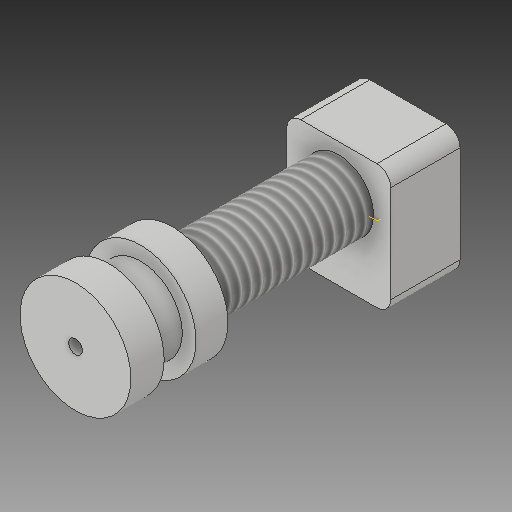
# Autodesk Inventor part: Hotend Mock Up
Saved by Autodesk Inventor 2018 (Build 220112000, 112)
## iProperties
Created: 2016-06-25
Part Number: Hotend Mock Up
Material: Generic
Document SubType Name: Modeling
Designer: joshm
Density: 1 g/cm^3
Appearance: Default
Mass: 6.93473 g
Surface Area: 30.5919 cm^2
Volume: 6.93473 cm^3
Author: joshm
Autodesk Inventor part; units mm, degrees
ref_plane "YZ Plane" through (0, 0, 0) normal (1, 0, 0) x (0, 1, 0)
ref_plane "XZ Plane" through (0, 0, 0) normal (0, 1, 0) x (-1, 0, 0)
ref_plane "XY Plane" through (0, 0, 0) normal (0, 0, 1) x (1, 0, 0)
sketch "Sketch1" plane through (0, 0, 0) normal (0, 0, 1) x (1, 0, 0)
  arc A0 (10.5041, 10) -> (25.996, 10) centre (18.25, 12) ccw projected
  circle A1 centre (18.25, 12) radius 8
  point P0 (0, 0)
  constraints: 1 centre point, 1 coincident, 1 concentric
extrude "Extrusion1" add sketch "Sketch1" against normal blind 4.8
sketch "Sketch2" plane through (18.25, 12, -4.8) normal (0, 0, -1) x (-1, 0, 0)
  circle A0 centre (0, 0) radius 8 projected
  circle A1 centre (0, 0) radius 6
  point P0 (18.25, -12)
  dimension "d2" = 12
  constraints: 1 centre point, 1 coincident
  measures "d2" diameter of A1
extrude "Extrusion2" add sketch "Sketch2" along normal blind 4.6 contours A1
sketch "Sketch3" plane through (18.25, 12, -9.4) normal (0, 0, -1) x (-1, 0, 0)
  circle A0 centre (0, 0) radius 6 projected
  circle A1 centre (0, 0) radius 8
  point P0 (18.25, -12)
  constraints: 1 centre point, 1 coincident
extrude "Extrusion3" add sketch "Sketch3" along normal blind 4.6 contours A0 | A1
sketch "Sketch4" plane through (18.25, 12, -14) normal (0, 0, -1) x (-1, 0, 0)
  circle A0 centre (0, 0) radius 8 projected
  circle A1 centre (0, 0) radius 5
  point P0 (18.25, -12)
  dimension "d7" = 10
  constraints: 1 centre point, 1 coincident
  measures "d7" diameter of A1
extrude "Extrusion4" add sketch "Sketch4" along normal blind 24 contours A1
thread "Thread1" size "M10x1.5" class "6g" standard "ANSI Metric M Profile" full length
sketch "Sketch5" plane through (18.25, 12, -38) normal (0, 0, -1) x (-1, 0, 0)
  line L0 (-5.5007, -11.3783) -> (5.4993, -11.3783)
  line L1 (7.4993, -9.3783) -> (7.4993, 4.6217)
  line L2 (5.4993, 6.6217) -> (-5.5007, 6.6217)
  line L3 (-7.5007, 4.6217) -> (-7.5007, -9.3783)
  line L4 (-7.5007, -11.3783) -> (7.4993, 6.6217) construction
  line L5 (7.4993, -11.3783) -> (-7.5007, 6.6217) construction
  arc A0 (7.4993, 4.6217) -> (5.4993, 6.6217) centre (5.4993, 4.6217) ccw
  arc A1 (-5.5007, 6.6217) -> (-7.5007, 4.6217) centre (-5.5007, 4.6217) ccw
  arc A2 (-7.5007, -9.3783) -> (-5.5007, -11.3783) centre (-5.5007, -9.3783) ccw
  arc A3 (5.4993, -11.3783) -> (7.4993, -9.3783) centre (5.4993, -9.3783) ccw
  point P0 (18.25, -12)
  point P1 (-0.0007, -2.3783)
  dimension "d12" = 15
  dimension "d13" = 18
  dimension "d14" = 2
  constraints: 12 end point, 8 point on circle, 8 point on line, 8 tangent, 4 centre point, 3 equal radius, 2 midpoint, 2 parallel, 1 horizontal, 1 perpendicular
  measures "d12" distance of L5.end L4.end
  measures "d13" distance of L4.end L5.start
  measures "d14" radius of A0
extrude "Extrusion5" add sketch "Sketch5" along normal blind 10
sketch "Sketch6" plane through (18.25, 12, -48) normal (0, 0, -1) x (-1, 0, 0)
  circle A0 centre (0, 0) radius 5 projected
  circle A1 centre (0, 0) radius 1.15
  point P0 (18.25, -12)
  dimension "d17" = 2.3
  constraints: 1 centre point, 1 coincident
  measures "d17" diameter of A1
ref_plane "Work Plane1" through (12.7508, 11.9997, -38) normal (0, 1, 0) x (1, 0, 0)
sketch "Sketch7" plane through (12.7508, 11.9997, -38) normal (0, 1, 0) x (1, 0, 0)
  line L0 (6.6493, 10) -> (4.3493, 10) projected
  line L1 (5.4993, 10) -> (5.4993, 14.106)
  line L2 (5.3539, 14.106) -> (4.3493, 10)
  line L3 (5.4993, 14.106) -> (5.3539, 14.106)
  line L4 (5.4993, 14.106) -> (5.6446, 14.106) construction
  line L5 (5.4993, 10) -> (4.3493, 10)
  line L6 (4.3493, 10) -> (5.3539, 14.106)
  point P0 (-12.7508, -38)
  dimension "d20" = 180
  constraints: 12 end point, 3 collinear, 1 horizontal, 1 vertical
  measures "d20" angle of L3 L4
revolve "Revolution1" add sketch "Sketch7" angle 360 about axis through (18.25, 11.9997, -48) along (0, 0, -1)
sketch "Sketch8" plane through (18.25, 11.9997, -52.106) normal (0, 0, -1) x (-1, 0, 0)
  circle A0 centre (0, 0) radius 0.1454 projected
  circle A1 centre (0, 0) radius 0.1
  point P0 (18.25, -11.9997)
  dimension "d22" = 0.2
  constraints: 1 centre point, 1 coincident
  measures "d22" diameter of A1
extrude "Extrusion6" cut sketch "Sketch8" against normal up to surface (4.106 mm away) contours A1
sketch "Sketch9" plane through (18.25, 12, -48) normal (0, 0, -1) x (-1, 0, 0)
  line L0 (2.1554, 3.8954) -> (0.7949, 3.8954)
  line L1 (0.7949, 3.8954) -> (0.7949, -1.2159)
  line L2 (0.7949, -1.2159) -> (2.1554, -1.2159)
  line L3 (2.1554, -1.2159) -> (2.1554, 3.8954)
  line L4 (2.1554, 3.8954) -> (0.7949, -1.2159) construction
  line L5 (0.7949, 3.8954) -> (2.1554, -1.2159) construction
  line L6 (-2.1285, 4.9618) -> (-0.8047, 4.9618)
  line L7 (-0.8047, 4.9618) -> (-0.8047, -1.2159)
  line L8 (-0.8047, -1.2159) -> (-2.1285, -1.2159)
  line L9 (-2.1285, -1.2159) -> (-2.1285, 4.9618)
  line L10 (-2.1285, 4.9618) -> (-0.8047, -1.2159) construction
  line L11 (-0.8047, 4.9618) -> (-2.1285, -1.2159) construction
  point P0 (18.25, -12)
  point P1 (1.4752, 1.3398)
  point P2 (-1.4666, 1.873)
  constraints: 24 end point, 4 midpoint, 4 parallel, 2 horizontal, 2 perpendicular, 1 point on line
extrude "Extrusion7" cut sketch "Sketch9" along normal blind 10
sketch "Sketch10" plane through (18.25, 12, 0) normal (0, 0, 1) x (1, 0, 0)
  circle A0 centre (0, 0) radius 8 projected
  point P0 (-18.25, -12)
  point P1 (0.8047, 0.8213)
hole "Hole1" at (18.25, 12, 0) direction (0, 0, -1) diameter 2 depth 10 tip angle 118
body "Solid1"
